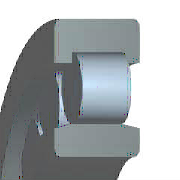
# Autodesk Inventor part: DIN 5412 T1 - NU1020 - 100 x 150 x 24
Saved by Autodesk Inventor 2026.2 (Build 302298010, 298A)
## iProperties
Created: 2025-01-21
Part Number: DIN 5412 T1 - NU1020 - 100 x 150 x 24
Material: Steel, Mild
Description: Cylindrical Roller Bearing
Document SubType Name: Modeling
Standard: DIN 5412 T1
Designer: Yan
Standard Revision: 2005-08
Standards Organization: DIN
Language: en-US
Size Designation: NU1020 - 100 x 150 x 24
Categories: <MemberInstance><Categories><Category DisplayName="Shaft Parts" InternalName="7f7aeb1f-a693-4053-b835-cee3144e0d98" Mnemonic="SHFT"><Category DisplayName="Bearings" InternalName="242d30a3-7172-44e6-a363-b0a3d8f1b556" Mnemonic="BRNG"><CategoryParameter DisplayName="Width" InternalName="25fc5f6e-338b-4801-b5ed-8959743e396e" Mnemonic="wdth"/><CategoryParameter DisplayName="Size Designation" InternalName="2c4e891a-c8f4-49ed-a5c1-5131476c6feb" Mnemonic="sizedes"/><CategoryParameter DisplayName="Basic Dynamic Load Rating" InternalName="440972dd-7009-4861-bd45-69ffbb461423" Mnemonic="bdynlrat"/><CategoryParameter DisplayName="Shaft Diameter" InternalName="91302473-2833-4451-a660-c5d4a8d6a031" Mnemonic="shaftdia"/><CategoryParameter DisplayName="Touch Angle" InternalName="aa21a452-7974-4a55-b5cf-1c2972de2aea" Mnemonic="TouchAngle"/><CategoryParameter DisplayName="Outer Diameter" InternalName="d441686c-04bd-4681-b674-94fbc173ec23" Mnemonic="outdia"/><Category DisplayName="Roller Bearings" InternalName="a40a3fd7-d489-4921-9892-cb944902a182" Mnemonic="ROLLBEAR"><CategoryParameter DisplayName="Basic Static Load Rating" InternalName="124ef669-bc53-497e-8b3b-9e9432584ac1" Mnemonic="bstatlrat"/><CategoryParameter DisplayName="Radial Dynamic Load Factor when Fa/Fr &gt; e" InternalName="1feec4eb-3d91-4913-989d-fa96ab069f3d" Mnemonic="raddynfc2"/><CategoryParameter DisplayName="Axial Dynamic Load Factor when Fa/Fr &gt; e" InternalName="200b4357-faba-40fb-9da6-9412c8ddeb78" Mnemonic="axdynfc2"/><CategoryParameter DisplayName="Radius" InternalName="2322b21e-a448-4b16-bf77-0b09a9a1e5fa" Mnemonic="rad"/><CategoryParameter DisplayName="Min. Shaft Diameter" InternalName="27c639de-1f82-42cb-a17a-a84ebe509f1b" Mnemonic="minshaftdia"/><CategoryParameter DisplayName="Limiting Speed Lubrication Grease" InternalName="34ed7782-22cd-44b7-90f2-16a4b10c8234" Mnemonic="lubgrsp"/><CategoryParameter DisplayName="Mass" InternalName="35563771-cdde-4f36-b8ea-a6490dc90073" Mnemonic="mass"/><CategoryParameter DisplayName="Limiting Speed Oil" InternalName="576744bc-a99a-4f12-bf8b-8b83672ef882" Mnemonic="oilspd"/><CategoryParameter DisplayName="Radial Static Load Factor" InternalName="646321f5-f93b-4aec-b962-0341aa1dcfaf" Mnemonic="raddynfc0"/><CategoryParameter DisplayName="Max. Step Fillet Radius" InternalName="890763e8-95b6-457a-9b07-8de657924e40" Mnemonic="maxstprad"/><CategoryParameter DisplayName="Axial Dynamic Load Factor when Fa/Fr &lt;= e" InternalName="b1d498d2-5149-4618-b12c-23a3d5a7c887" Mnemonic="axdynfc1"/><CategoryParameter DisplayName="Radial Dynamic Load Factor when Fa/Fr &lt;= e" InternalName="b75e8b40-fb1d-483d-887b-ce2ffe1b5422" Mnemonic="raddynfc1"/><CategoryParameter DisplayName="Friction Factor" InternalName="ceddb76f-d381-429d-bef5-367584929fdf" Mnemonic="fricfct"/><CategoryParameter DisplayName="Axial Static Load Factor" InternalName="ea413b62-e115-405b-882c-23d570c3be21" Mnemonic="axdynfc0"/><CategoryParameter DisplayName="Limiting Value for Factor Determination" InternalName="f0539972-a230-481a-8ae0-28002199c8fb" Mnemonic="limvalfac"/><CategoryParameter DisplayName="Exponent for Determining Life" InternalName="f80a4cc4-8fb3-4eaa-808e-6f490e608712" Mnemonic="lifeexp"/><CategoryParameter DisplayName="Max. Hub Step Diameter" InternalName="feeea31f-2614-4692-af6e-a054e6e558b2" Mnemonic="maxhubdia"/><Category DisplayName="Cylindrical Roller Bearings" InternalName="e9f1187d-0783-4354-b25c-5013db6f4580" Mnemonic="RBCRB"/></Category></Category></Category><Category DisplayName="DataType" InternalName="23b78d0f-2648-40c6-8793-ca6db495c9e8" Mnemonic="DATATYPE"><CategoryParameter DisplayName="DisplayName" InternalName="05415f3d-3907-474b-a020-eb9d644f4cf3" Mnemonic="DISPLAYNAME"/><CategoryParameter DisplayName="Standard" InternalName="0c0a119c-1e12-4c84-803f-101930972f5e" Mnemonic="STANDARD"/><CategoryParameter DisplayName="Description" InternalName="13903e3d-64b1-4950-80da-f627842ea37f" Mnemonic="DESCRIPTION"/><CategoryParameter DisplayName="Designation" InternalName="2675968c-4ce5-49e0-a4f5-552d29089031" Mnemonic="DESIGNATION"/><CategoryParameter DisplayName="Default Row" InternalName="2af9ec52-faaa-4026-b378-f9fa4afca842" Mnemonic="DEFAULTROW"/><CategoryParameter DisplayName="Folder Name" InternalName="3f06958e-8713-4116-9be7-ed6184ecc97b" Mnemonic="FOLDERNAME"/><CategoryParameter DisplayName="Revision Guid" InternalName="45a75005-10b1-4dfc-8d6d-dfe629f0b93c" Mnemonic="REVISIONGUID"/><CategoryParameter DisplayName="FileName" InternalName="8b46a4cc-9585-4fed-90c3-899f57e09a73" Mnemonic="FILENAME"/><CategoryParameter DisplayName="StdsOrg" InternalName="8f5914e1-4693-403f-8ab5-d37768198c9d" Mnemonic="STDSORG"/><CategoryParameter DisplayName="Family Version" InternalName="914462f6-6e19-4b14-ba84-155b9680b1d0" Mnemonic="FAMILYREVISION"/><CategoryParameter DisplayName="Standard Revision" InternalName="91d5a463-65c2-4fde-b823-3b7fea5e8e17" Mnemonic="STANDARDREVISION"/><CategoryParameter DisplayName="Member Revision" InternalName="a65d44b9-392f-4f4f-857b-e4b3d54996fe" Mnemonic="MEMBERREVISION"/><CategoryParameter DisplayName="ClipFormat" InternalName="bc51e27b-3422-4e78-93ef-cec197ddf230" Mnemonic="CLIPFORMAT"/><CategoryParameter DisplayName="Manufacturer" InternalName="cd6c7a72-a28a-4e50-99a9-2c7f4e13e5ad" Mnemonic="MANUFACTURER"/><CategoryParameter DisplayName="InternalName" InternalName="cf1d0246-76d9-4b4a-8305-fa0409afb5c1" Mnemonic="INTERNALNAME"/><CategoryParameter DisplayName="IsMetric" InternalName="e2385c5b-1ea4-4823-96a8-8de651266ec3" Mnemonic="ISMETRIC"/><Category DisplayName="Part" InternalName="c0e0b642-3bcb-4cc8-9e80-f96d35c4afa4" Mnemonic="PART"><CategoryParameter DisplayName="Part Number" InternalName="016b6077-bfbe-49bd-92c9-d8d59c39c941" Mnemonic="PARTNUMBER"/><CategoryParameter DisplayName="Stock Number" InternalName="4dba7c1c-e26c-444e-836c-b08b433409a8" Mnemonic="STOCKNUMBER"/><CategoryParameter DisplayName="Material Key" InternalName="5c9a8adb-dd2b-4535-b97f-0a94a95fe41f" Mnemonic="MATERIALKEY"/><CategoryParameter DisplayName="Material" InternalName="818a152a-d3c3-49ca-80ee-df7d91421b8e" Mnemonic="MATERIAL"/></Category></Category><Category DisplayName="LegacyMap" InternalName="cd87c42b-3e48-431e-b5c0-1cbeb14dfe77" Mnemonic="LEGACYMAP"><CategoryParameter DisplayName="unique DA member ID" InternalName="0918ad47-427f-4fed-ae26-24c81c58f590" Mnemonic="DACOOKIE"/><CategoryParameter DisplayName="Merge11 ID" InternalName="0ee8fb18-e2ed-4f39-96f6-1f4b5f50aa71" Mnemonic="MERGE11"/><CategoryParameter DisplayName="unique CC member ID" InternalName="5193edd4-b2b0-4ab4-9d54-de900eee34e0" Mnemonic="CCCOOKIE"/><CategoryParameter DisplayName="Split ID" InternalName="72b5c83c-be7f-45c4-ae51-9160ea6deb26" Mnemonic="SPLIT"/><CategoryParameter DisplayName="MemberID" InternalName="8e5e0294-fc51-4c8f-b3d7-003dc5ed94f6" Mnemonic="MEMBERID"/><CategoryParameter DisplayName="CatalogName" InternalName="d99d1e27-aa94-4de2-af4c-c348882a6f4f" Mnemonic="CATALOGNAME"/><CategoryParameter DisplayName="FamilyNumber" InternalName="e705e1f4-09cb-413e-91f9-551b4188271e" Mnemonic="FAMILYNUMBER"/></Category></Categories><FamilyTemplate Id="br0023"><FamilyTemplateParameters><FamilyTemplateParameter ObjectType="kUserParameterObject" ValueType="xs:double" Id="1" ObjectReferenceKey="ACA"/><FamilyTemplateParameter ObjectType="kUserParameterObject" ValueType="xs:double" Id="2" ObjectReferenceKey="WR"/><FamilyTemplateParameter ObjectType="kUserParameterObject" ValueType="xs:double" Id="3" ObjectReferenceKey="BC"/><FamilyTemplateParameter ObjectType="kUserParameterObject" ValueType="xs:double" Id="4" ObjectReferenceKey="KR1S"/><FamilyTemplateParameter ObjectType="kUserParameterObject" ValueType="xs:double" Id="5" ObjectReferenceKey="KRS"/><FamilyTemplateParameter ObjectType="kUserParameterObject" ValueType="xs:double" Id="6" ObjectReferenceKey="WD"/><FamilyTemplateParameter ObjectType="kUserParameterObject" ValueType="xs:double" Id="7" ObjectReferenceKey="KAD1"/><FamilyTemplateParameter ObjectType="kUserParameterObject" ValueType="xs:double" Id="8" ObjectReferenceKey="KB"/><FamilyTemplateParameter ObjectType="kUserParameterObject" ValueType="xs:double" Id="9" ObjectReferenceKey="BBA"/><FamilyTemplateParameter ObjectType="kUserParameterObject" ValueType="xs:double" Id="10" ObjectReferenceKey="BC0"/><FamilyTemplateParameter ObjectType="kUserParameterObject" ValueType="xs:double" Id="11" ObjectReferenceKey="BD"/><FamilyTemplateParameter ObjectType="kUserParameterObject" ValueType="xs:double" Id="12" ObjectReferenceKey="BR"/><FamilyTemplateParameter ObjectType="kUserParameterObject" ValueType="xs:double" Id="13" ObjectReferenceKey="DDB"/><FamilyTemplateParameter ObjectType="kUserParameterObject" ValueType="xs:double" Id="14" ObjectReferenceKey="KID1"/><FamilyTemplateParameter ObjectType="kUserParameterObject" ValueType="xs:double" Id="15" ObjectReferenceKey="BI"/><FamilyTemplateParameter ObjectType="kPropertyObject" ValueType="xs:string" Id="100" ObjectReferenceKey="{32853F0F-3444-11d1-9E93-0060B03C1CA6}" SubObjectId="52"/><FamilyTemplateParameter ObjectType="kPropertyObject" ValueType="xs:string" Id="105" ObjectReferenceKey="{32853F0F-3444-11d1-9E93-0060B03C1CA6}" SubObjectId="5"/><FamilyTemplateParameter ObjectType="kPartComponentDefinitionObject" ValueType="xs:string" Id="110" SubObjectId="Material"/></FamilyTemplateParameters></FamilyTemplate><CategoryParameterMap><ParamToTemplateMap><ParamToTemplate CategoryParameter="//CategoryParameter[@InternalName='05415f3d-3907-474b-a020-eb9d644f4cf3']" ConstantValue="DIN 5412 - T1 NU"/><ParamToTemplate CategoryParameter="//CategoryParameter[@InternalName='cf1d0246-76d9-4b4a-8305-fa0409afb5c1']" ConstantValue="15f18d82-9a5a-48ed-96ca-9b0d6c7c2b54"/><ParamToTemplate CategoryParameter="//CategoryParameter[@InternalName='3f06958e-8713-4116-9be7-ed6184ecc97b']" ConstantValue="DIN 5412 - T1  NU"/><ParamToTemplate CategoryParameter="//CategoryParameter[@InternalName='914462f6-6e19-4b14-ba84-155b9680b1d0']" ConstantValue="10"/><ParamToTemplate CategoryParameter="//CategoryParameter[@InternalName='bc51e27b-3422-4e78-93ef-cec197ddf230']" ConstantValue="CF_INVENTOR.STDPARTS"/><ParamToTemplate CategoryParameter="//CategoryParameter[@InternalName='e2385c5b-1ea4-4823-96a8-8de651266ec3']" ConstantValue="true"/><ParamToTemplate CategoryParameter="//CategoryParameter[@InternalName='13903e3d-64b1-4950-80da-f627842ea37f']" ConstantValue="Cylindrical Roller Bearing"/><ParamToTemplate CategoryParameter="//CategoryParameter[@InternalName='8f5914e1-4693-403f-8ab5-d37768198c9d']" ConstantValue="DIN"/><ParamToTemplate CategoryParameter="//CategoryParameter[@InternalName='0c0a119c-1e12-4c84-803f-101930972f5e']" ConstantValue="DIN 5412 T1"/><ParamToTemplate CategoryParameter="//CategoryParameter[@InternalName='cd6c7a72-a28a-4e50-99a9-2c7f4e13e5ad']" TemplateParameter="104"/><ParamToTemplate CategoryParameter="//CategoryParameter[@InternalName='91d5a463-65c2-4fde-b823-3b7fea5e8e17']" ConstantValue="2005-08"/><ParamToTemplate CategoryParameter="//CategoryParameter[@InternalName='45a75005-10b1-4dfc-8d6d-dfe629f0b93c']" ConstantValue="b3ce8b6f-dbef-4b1d-b0ff-74675c80c21c"/><ParamToTemplate CategoryParameter="//CategoryParameter[@InternalName='2af9ec52-faaa-4026-b378-f9fa4afca842']" ConstantValue="10"/><ParamToTemplate CategoryParameter="//CategoryParameter[@InternalName='d99d1e27-aa94-4de2-af4c-c348882a6f4f']" ConstantValue="DIN"/><ParamToTemplate CategoryParameter="//CategoryParameter[@InternalName='e705e1f4-09cb-413e-91f9-551b4188271e']" ConstantValue="260"/><ParamToTemplate CategoryParameter="//CategoryParameter[@InternalName='8b46a4cc-9585-4fed-90c3-899f57e09a73']" ConstantValue="DIN 5412 T1 - NU1020 - 100 x 150 x 24"/><ParamToTemplate CategoryParameter="//CategoryParameter[@InternalName='a65d44b9-392f-4f4f-857b-e4b3d54996fe']" ConstantValue="F92977C2-9FF2-44BC-AD25-3305368DF2CF"/><ParamToTemplate CategoryParameter="//CategoryParameter[@InternalName='2c4e891a-c8f4-49ed-a5c1-5131476c6feb']" ConstantValue="NU1020"/><ParamToTemplate CategoryParameter="//CategoryParameter[@InternalName='8e5e0294-fc51-4c8f-b3d7-003dc5ed94f6']" ConstantValue="1770"/><ParamToTemplate CategoryParameter="//CategoryParameter[@InternalName='aa21a452-7974-4a55-b5cf-1c2972de2aea']" TemplateParameter="9"/><ParamToTemplate CategoryParameter="//CategoryParameter[@InternalName='440972dd-7009-4861-bd45-69ffbb461423']" TemplateParameter="3"/><ParamToTemplate CategoryParameter="//CategoryParameter[@InternalName='124ef669-bc53-497e-8b3b-9e9432584ac1']" TemplateParameter="10"/><ParamToTemplate CategoryParameter="//CategoryParameter[@InternalName='d441686c-04bd-4681-b674-94fbc173ec23']" TemplateParameter="11"/><ParamToTemplate CategoryParameter="//CategoryParameter[@InternalName='2675968c-4ce5-49e0-a4f5-552d29089031']" TemplateParameter="100"/><ParamToTemplate CategoryParameter="//CategoryParameter[@InternalName='25fc5f6e-338b-4801-b5ed-8959743e396e']" TemplateParameter="8"/><ParamToTemplate CategoryParameter="//CategoryParameter[@InternalName='2322b21e-a448-4b16-bf77-0b09a9a1e5fa']" TemplateParameter="5"/><ParamToTemplate CategoryParameter="//CategoryParameter[@InternalName='818a152a-d3c3-49ca-80ee-df7d91421b8e']" TemplateParameter="110"/><ParamToTemplate CategoryParameter="//CategoryParameter[@InternalName='016b6077-bfbe-49bd-92c9-d8d59c39c941']" TemplateParameter="105"/><ParamToTemplate CategoryParameter="//CategoryParameter[@InternalName='91302473-2833-4451-a660-c5d4a8d6a031']" TemplateParameter="6"/></ParamToTemplateMap></CategoryParameterMap></MemberInstance>
Density: 7.85 g/cm^3
Appearance: Semi-Polished
IsCustomPart: 0
Author: Yan
Autodesk Inventor part; units mm, degrees
ref_plane "YZ Plane" through (0, 0, 0) normal (1, 0, 0) x (0, 1, 0)
ref_plane "XZ Plane" through (0, 0, 0) normal (0, 1, 0) x (-1, 0, 0)
ref_plane "XY Plane" through (0, 0, 0) normal (0, 0, 1) x (1, 0, 0)
sketch "Sketch" plane through (0, 0, 0) normal (0, 0, 1) x (1, 0, 0)
  line L0 (4.8, 69) -> (19.2, 69)
  line L1 (19.2, 69) -> (19.2, 56.5)
  line L2 (19.2, 56.5) -> (4.8, 56.5)
  line L3 (4.8, 56.5) -> (4.8, 69)
  line L4 (19.2, 62.75) -> (4.8, 62.75)
  line L5 (4.8, 66.25) -> (0, 66.25)
  line L6 (12, 62.75) -> (12, 56.5)
  line L7 (4.8, 56.5) -> (0, 55.65363)
  line L8 (0, 50) -> (24, 50)
  line L9 (0, 75) -> (24, 75)
  line L10 (19.2, 56.5) -> (19.2, 69)
  line L11 (19.2, 66.25) -> (24, 66.25)
  line L12 (19.2, 56.5) -> (24, 55.65363)
  line L13 (24, 50) -> (24, 55.65363)
  line L14 (24, 66.25) -> (24, 75)
  line L15 (-4.4, 0) -> (26.4, 0)
  line L16 (0, -1.7) -> (0, 11.95)
  dimension "d0" = 10
  dimension "d12" = 100
  dimension "d13" = 113
  dimension "d14" = 132.5
  dimension "d15" = 150
  dimension "d16" = 138
  dimension "d17" = 4.8
  dimension "d18" = 24
  constraints: 30 end point, 6 point on line, 4 midpoint, 4 symmetric about line, 3 parallel, 2 perpendicular, 1 horizontal, 3 other
  measures "d0" angle of L8 L7
  measures "d12" diameter of L8 L15
  measures "d13" diameter of L2 L15
  measures "d14" diameter of L5 L15
  measures "d15" diameter of L9 L15
  measures "d16" diameter of L0 L15
  measures "d17" distance between parallel lines of L16 L3
  measures "d18" distance between parallel lines of L16 L13
sketch "Sketch outline for Body" plane through (0, 0, 0) normal (0, 0, 1) x (1, 0, 0)
  line L0 (24, 55.65363) -> (19.2, 56.5)
  line L1 (19.2, 56.5) -> (4.8, 56.5)
  line L2 (4.8, 56.5) -> (0, 55.65363)
  line L3 (0, 55.65363) -> (0, 50)
  line L4 (0, 50) -> (24, 50)
  line L5 (24, 50) -> (24, 55.65363)
  line L6 (4.8, 66.25) -> (4.8, 69)
  line L7 (0, 66.25) -> (4.8, 66.25)
  line L8 (0, 75) -> (0, 66.25)
  line L9 (24, 75) -> (0, 75)
  line L10 (24, 66.25) -> (24, 75)
  line L11 (19.2, 66.25) -> (24, 66.25)
  line L12 (19.2, 69) -> (19.2, 66.25)
  line L13 (4.8, 69) -> (19.2, 69)
revolve "Body" add sketch "Sketch outline for Body" angle 360 about axis through (-10, 0, 0) along (1, 0, 0)
fillet "Fillet1" radius 1.1 2 edges at (24, -75, 0) (0, -75, 0)
fillet "Fillet1" radius 1.5 2 edges at (0, -50, 0) (24, -50, 0)
revolve "Roller" add sketch "Sketch" angle 360 about axis through (19.2, 62.75, 0) along (-1, 0, 0) contours L0 L1 L4 L3
pattern_circular "Rollers" count 16 over 360 about axis through (-10, 0, 0) along (1, 0, 0) of "Roller"
equation "\"d12\" = WD"
equation "\"d13\" = KID1"
equation "\"d14\" = KAD1"
equation "\"d15\" = BD"
equation "\"d16\" = KID1 + 2 * DDB"
equation "\"d17\" = ACA"
equation "\"d18\" = KB"
equation "\"d3\" = KR1S"
equation "\"d4\" = KRS"
equation "\"WD\" = 100"
equation "\"BD\" = 150"
equation "\"KB\" = 24"
equation "\"KAD1\" = 0.5 * BD + 0.5 * WD + 0.6 * DDB"
equation "\"KID1\" = 113"
equation "\"KRS\" = 1.5"
equation "\"KR1S\" = 1.1"
equation "\"DDB\" = -0.25 * WD + 0.25 * BD"
equation "\"ACA\" = 0.2 * KB"
equation "\"BBA\" = 0"
equation "\"BR\" = 0.5 * BD"
body "Solid1"
